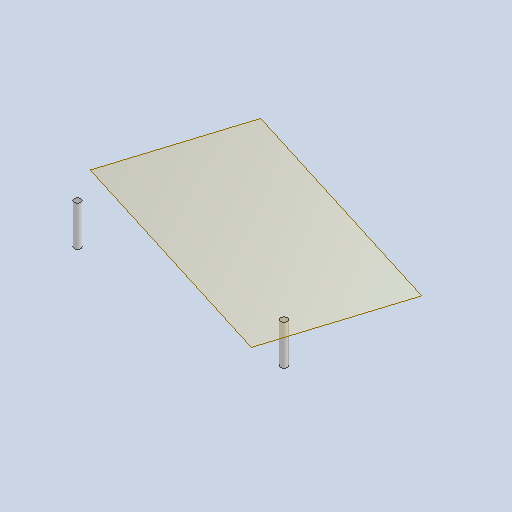
# Autodesk Inventor part: fitting
Saved by Autodesk Inventor 2025.1 (Build 291241000, 241)
## iProperties
Created: 2024-09-13
Part Number: fitting
Material: Generic
Document SubType Name: Modeling
Designer: ffogue
Density: 1 g/cm^3
Appearance: Default
Author: ffogue
Autodesk Inventor part; units mm, degrees
ref_plane "YZ Plane" through (0, 0, 0) normal (1, 0, 0) x (0, 1, 0)
ref_plane "XZ Plane" through (0, 0, 0) normal (0, 1, 0) x (-1, 0, 0)
ref_plane "XY Plane" through (0, 0, 0) normal (0, 0, 1) x (1, 0, 0)
sketch "Sketch1" plane through (0, 0, 0) normal (0, 0, 1) x (1, 0, 0)
  circle A0 centre (62, -18.6078) radius 2 projected
  point P0 (0, 0)
extrude "Extrusion1" add sketch "Sketch1" against normal blind 24
ref_plane "Work Plane1" through (8.3649, 17.6348, 0) normal (0, 0, 1) x (0.9545, -0.2981, 0)
sketch "Sketch2" plane through (8.3649, 17.6348, 0) normal (0, 0, 1) x (0.9545, -0.2981, 0)
  circle A0 centre (-56.3633, -55.5691) radius 2 projected
  point P0 (-2.7282, -19.3265)
extrude "Extrusion2" add sketch "Sketch2" against normal blind 24
body "Solid1"
